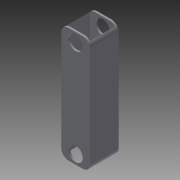
# Autodesk Inventor part: 4inLink
Saved by Autodesk Inventor 2014 (Build 180170000, 170)
## iProperties
Created: 2016-01-10
Part Number: 4inLink
Material: Generic
Document SubType Name: Modeling
Designer: Applefamily
Density: 1 g/cm^3
Appearance: Default
Author: Applefamily
Autodesk Inventor part; units mm, degrees
ref_plane "YZ Plane" through (0, 0, 0) normal (1, 0, 0) x (0, 1, 0)
ref_plane "XZ Plane" through (0, 0, 0) normal (0, 1, 0) x (-1, 0, 0)
ref_plane "XY Plane" through (0, 0, 0) normal (0, 0, 1) x (1, 0, 0)
sketch "Sketch1" plane through (0, 0, 0) normal (0, 1, 0) x (-1, 0, 0)
  line L0 (-6.7886, -4.7076) -> (18.6114, -4.7076)
  line L1 (18.6114, -4.7076) -> (18.6114, 20.6924)
  line L2 (18.6114, 20.6924) -> (-6.7886, 20.6924)
  line L3 (-6.7886, 20.6924) -> (-6.7886, -4.7076)
  line L4 (-5.2011, -3.1201) -> (17.0239, -3.1201)
  line L5 (17.0239, -3.1201) -> (17.0239, 19.1049)
  line L6 (17.0239, 19.1049) -> (-5.2011, 19.1049)
  line L7 (-5.2011, 19.1049) -> (-5.2011, -3.1201)
  point P0 (0, 0)
  dimension "d0" = 25.4
  dimension "d1" = 25.4
  dimension "d2" = 1.5875
  dimension "d3" = 1.5875
  dimension "d4" = 1.5875
  dimension "d5" = 1.5875
  constraints: 16 end point, 4 parallel, 2 horizontal, 2 perpendicular
  measures "d0" distance of L2.end L1.end
  measures "d1" distance of L1.end L0.end
  measures "d2" horizontal distance of L4.start L0.start
  measures "d3" horizontal distance of L4.end L0.end
  measures "d4" horizontal distance of L1.end L5.end
  measures "d5" horizontal distance of L2.end L6.end
extrude "Extrusion1" add sketch "Sketch1" along normal blind 101.6
sketch "Sketch2" plane through (-18.6114, 0, 20.6924) normal (0, 0, 1) x (1, 0, 0)
  circle A0 centre (12.7, 8.255) radius 6.35
  circle A1 centre (12.7, 93.345) radius 6.35
  point P0 (25.4, 0)
  point P1 (25.4, 101.6)
  point P2 (18.6114, 0)
  dimension "d8" = 12.7
  dimension "d9" = 12.7
  dimension "d10" = 8.255
  dimension "d11" = 8.255
  constraints: 2 centre point
  measures "d8" diameter of A0
  measures "d9" diameter of A1
  measures "d10" vertical distance of A0.centre point (25.4, 0)
  measures "d11" vertical distance of point (25.4, 101.6) A1.centre
extrude "Extrusion2" cut sketch "Sketch2" against normal blind 101.6
fillet "Fillet1" radius 6.35 1 edges at (6.7886, 101.6, 7.9924)
fillet "Fillet2" radius 6.35 3 edges at (-18.6114, 101.6, 7.9924) (6.7886, 0, 7.9924) (-18.6114, 0, 7.9924)
equation "\"d3\" = d2"
equation "\"d4\" = d2"
equation "\"d5\" = d2"
equation "\"d11\" = d10"
body "Solid1"
